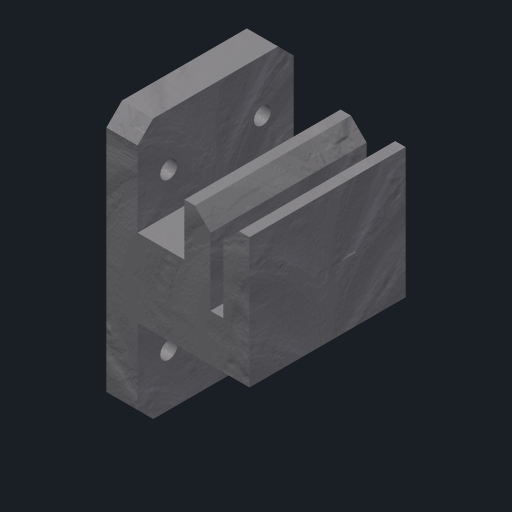
# Autodesk Inventor part: SEGURO
Saved by Autodesk Inventor 2024.3 (Build 283343000, 343)
## iProperties
Created: 2024-07-05
Part Number: SEGURO
Material: Steel, Mild, Welded
Document SubType Name: Modeling
Designer: Niler
Density: 7.85 g/cm^3
Appearance: Weld - Steel Mild
Author: Niler
Autodesk Inventor part; units mm, degrees
ref_plane "YZ Plane" through (0, 0, 0) normal (1, 0, 0) x (0, 1, 0)
ref_plane "XZ Plane" through (0, 0, 0) normal (0, 1, 0) x (-1, 0, 0)
ref_plane "XY Plane" through (0, 0, 0) normal (0, 0, 1) x (1, 0, 0)
sketch "Sketch1" plane through (0, 0, 0) normal (1, 0, 0) x (0, 1, 0)
  line L0 (-25, 15) -> (25, 15)
  line L1 (25, 15) -> (25, -15)
  line L2 (25, -15) -> (-25, -15)
  line L3 (-25, -15) -> (-25, 15)
  line L4 (-25, 15) -> (25, -15) construction
  line L5 (25, 15) -> (-25, -15) construction
  line L6 (-15, -9) -> (15, -9) construction
  line L7 (15, -9) -> (15, 9) construction
  line L8 (15, 9) -> (-15, 9) construction
  line L9 (-15, 9) -> (-15, -9) construction
  line L10 (-15, -9) -> (15, 9) construction
  line L11 (15, -9) -> (-15, 9) construction
  circle A0 centre (15, -9) radius 1.65
  circle A1 centre (15, 9) radius 1.65
  circle A2 centre (-15, 9) radius 1.65
  circle A3 centre (-15, -9) radius 1.65
  point P0 (0, 0)
  dimension "d0" = 50
  dimension "d1" = 30
  dimension "d4" = 30
  dimension "d5" = 3.3
  constraints: 24 end point, 4 centre point, 4 coincident, 4 midpoint, 4 parallel, 3 equal radius, 2 horizontal, 2 perpendicular, 1 point on line
  measures "d0" distance of L1.end L2.end
  measures "d1" distance of L0.end L1.end
  measures "d4" distance of L7.end L8.end
  measures "d5" diameter of A0
extrude "Extrusion1" add sketch "Sketch1" against normal blind 6
sketch "Sketch2" plane through (0, 0, 0) normal (1, 0, 0) x (0, 0, -1)
  line L0 (15, -25) -> (15, 25) projected
  line L1 (15, 25) -> (-15, 25) projected
  line L2 (-15, 25) -> (-15, -25) projected
  line L3 (-15, -25) -> (15, -25) projected
  circle A0 centre (9, -15) radius 1.65 projected
  circle A1 centre (-9, -15) radius 1.65 projected
  circle A2 centre (-9, 15) radius 1.65 projected
  circle A3 centre (9, 15) radius 1.65 projected
  line L4 (-15, -7.5) -> (15, -7.5)
  line L5 (15, -7.5) -> (15, 7.5)
  line L6 (15, 7.5) -> (-15, 7.5)
  line L7 (-15, 7.5) -> (-15, -7.5)
  line L8 (-15, -7.5) -> (15, 7.5) construction
  line L9 (15, -7.5) -> (-15, 7.5) construction
  point P0 (0, 0)
  point P1 (-15, 7.5)
  point P2 (-15, -7.5)
  dimension "d6" = 15
  constraints: 12 end point, 2 midpoint, 2 parallel, 1 horizontal, 1 perpendicular, 1 point on line
  measures "d6" distance between parallel lines of L4 L6
extrude "Extrusion2" add sketch "Sketch2" along normal blind 9 contours L4 L2 L6 L0
sketch "Sketch3" plane through (9, 0, 0) normal (1, 0, 0) x (0, 0, -1)
  line L0 (-15, 7.5) -> (-15, -7.5) projected
  line L1 (-15, -7.5) -> (15, -7.5) projected
  line L2 (15, -7.5) -> (15, 7.5) projected
  line L3 (15, 7.5) -> (-15, 7.5) projected
  line L4 (-15, -7.5) -> (15, -7.5)
  line L5 (15, -7.5) -> (15, 17.5)
  line L6 (15, 17.5) -> (-15, 17.5)
  line L7 (-15, 17.5) -> (-15, -7.5)
  point P0 (0, 0)
  dimension "d9" = 25
  constraints: 8 end point, 2 parallel, 1 horizontal, 1 perpendicular
  measures "d9" distance of L1.end L5.end
extrude "Extrusion3" add sketch "Sketch3" along normal blind 5
sketch "Sketch4" plane through (14, 0, 0) normal (1, 0, 0) x (0, 0, -1)
  line L0 (-15, 7.5) -> (15, 7.5) projected
  line L1 (15, 7.5) -> (-15, 7.5) projected
  line L2 (-15, -7.5) -> (15, -7.5) projected
  line L3 (15, -7.5) -> (15, 17.5) projected
  line L4 (15, 17.5) -> (-15, 17.5) projected
  line L5 (-15, 17.5) -> (-15, -7.5) projected
  point P0 (0, 0)
  point P1 (15, 7.5)
  point P2 (-15, 7.5)
extrude "Extrusion4" add sketch "Sketch4" along normal blind 2.5 contours L0 L3 L2 L5
sketch "Sketch5" plane through (16.5, 0, 0) normal (1, 0, 0) x (0, 0, -1)
  line L0 (-15, 7.5) -> (15, 7.5) projected
  line L1 (15, 7.5) -> (15, 17.5) projected
  line L2 (15, 17.5) -> (-15, 17.5) projected
  line L3 (-15, 17.5) -> (-15, 7.5) projected
  line L4 (15, -7.5) -> (15, 7.5) projected
  line L5 (15, 7.5) -> (-15, 7.5) projected
  line L6 (-15, 7.5) -> (-15, -7.5) projected
  line L7 (-15, -7.5) -> (15, -7.5) projected
  point P0 (0, 0)
extrude "Extrusion5" add sketch "Sketch5" along normal blind 5
chamfer "Chamfer1" distance 3 angle 45 2 edges at (14, 17.5, 0) (16.5, 17.5, 0)
sketch "Sketch6" plane through (14, 7.5, 15) normal (0, 1, 0) x (1, 0, 0)
  line L0 (0, 0) -> (0, 30) projected
  line L1 (0, 0) -> (2.5, 0) projected
  line L2 (2.5, 30) -> (2.5, 0) projected
  line L3 (0, 30) -> (2.5, 30) projected
  point P0 (-14, 15)
extrude "Extrusion6" cut sketch "Sketch6" against normal blind 6
chamfer "Chamfer2" distance 3 angle 45 4 edges at (-3, 25, 15) (-3, 25, -15) (-3, -25, -15) (-3, -25, 15)
body "Solid1"
